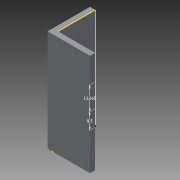
# Autodesk Inventor part: printed Y rod holder bracket
Saved by Autodesk Inventor 2014 SP1 (Build 180222100, 222)
## iProperties
Created: 2014-10-01
Part Number: printed Y rod holder bracket
Material: Generic
Document SubType Name: Modeling
Designer: Mon
Density: 1 g/cm^3
Appearance: Default
Author: Mon
Autodesk Inventor part; units mm, degrees
ref_plane "YZ Plane" through (0, 0, 0) normal (1, 0, 0) x (0, 1, 0)
ref_plane "XZ Plane" through (0, 0, 0) normal (0, 1, 0) x (-1, 0, 0)
ref_plane "XY Plane" through (0, 0, 0) normal (0, 0, 1) x (1, 0, 0)
sketch "Sketch1" plane through (0, 0, 0) normal (0, 0, 1) x (1, 0, 0)
  line L0 (0, 0) -> (25, 0)
  line L1 (25, 0) -> (25, 3)
  line L2 (25, 3) -> (3, 3)
  line L3 (3, 3) -> (3, 25)
  line L4 (3, 25) -> (0, 25)
  line L5 (0, 25) -> (0, 0)
  dimension "d0" = 25
  dimension "d1" = 3
  dimension "d2" = 22
  dimension "d3" = 22
  constraints: 12 end point, 4 parallel, 1 horizontal, 1 perpendicular
  measures "d0" distance of L0.start L0.end
  measures "d1" distance of L0.end L1.end
  measures "d2" distance of L1.end L2.end
  measures "d3" distance of L2.end L3.end
extrude "Extrusion1" add sketch "Sketch1" along normal blind 60
sketch "Sketch2" plane through (3, 3, 0) normal (1, 0, 0) x (0, 0, -1)
  line L0 (0, 0) -> (0, 22) projected
  line L1 (0, 22) -> (-60, 22) projected
  line L2 (-60, 0) -> (-60, 22) projected
  line L3 (0, 0) -> (-60, 0) projected
  line L4 (0, 22) -> (-1.4085, 22)
  line L5 (0, 22) -> (-9.5, 22) construction
  line L6 (-9.5, 22) -> (-8.5825, 22) construction
  line L7 (-9.5, 22) -> (-23.165, 22) construction
  line L8 (-23.165, 22) -> (-23.165, 2.4653) construction
  point P0 (0, -3)
  dimension "d6" = 9.5
  dimension "d7" = 13.665
  constraints: 10 end point, 4 point on line, 1 perpendicular
  measures "d6" distance of L0.end L5.end
  measures "d7" distance of L5.end L7.end
body "Solid1"
